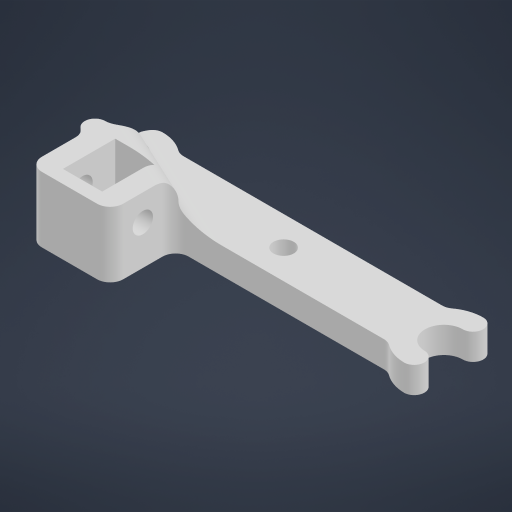
# Autodesk Inventor part: BaseMount
Saved by Autodesk Inventor 2023 (Build 270158000, 158)
## iProperties
Created: 2023-03-14
Part Number: BaseMount
Material: Generic
Document SubType Name: Modeling
Designer: Matt
Density: 1 g/cm^3
Appearance: Default
Author: Matt
Autodesk Inventor part; units mm, degrees
ref_plane "YZ Plane" through (0, 0, 0) normal (1, 0, 0) x (0, 1, 0)
ref_plane "XZ Plane" through (0, 0, 0) normal (0, 1, 0) x (-1, 0, 0)
ref_plane "XY Plane" through (0, 0, 0) normal (0, 0, 1) x (1, 0, 0)
sketch "Sketch1" plane through (0, 0, 0) normal (0, 1, 0) x (-1, 0, 0)
  circle A0 centre (0, 0) radius 2.4868
  line L0 (2.8868, 0) -> (1.4434, 2.5)
  line L1 (1.4434, 2.5) -> (-1.4434, 2.5)
  line L2 (-1.4434, 2.5) -> (-2.8868, 0)
  line L3 (-2.8868, 0) -> (-1.4434, -2.5)
  line L4 (-1.4434, -2.5) -> (1.4434, -2.5)
  line L5 (1.4434, -2.5) -> (2.8868, 0)
  line L6 (0, 0) -> (-23.467, 0)
  circle A1 centre (-49, 0) radius 2.4868
  line L7 (-46.1132, 0) -> (-47.5566, 2.5)
  line L8 (-47.5566, 2.5) -> (-50.4434, 2.5)
  line L9 (-50.4434, 2.5) -> (-51.8868, 0)
  line L10 (-51.8868, 0) -> (-50.4434, -2.5)
  line L11 (-50.4434, -2.5) -> (-47.5566, -2.5)
  line L12 (-47.5566, -2.5) -> (-46.1132, 0)
  arc A2 (43.788, 27) -> (35.788, 35) centre (35.788, 27) ccw
  line L13 (35.788, 35) -> (-48.212, 35)
  arc A3 (-48.212, 35) -> (-56.212, 27) centre (-48.212, 27) ccw
  line L14 (-56.212, 27) -> (-56.212, -62.0882)
  arc A4 (-56.212, -62.0882) -> (-54.3404, -67.2305) centre (-48.212, -62.0882) ccw
  line L15 (-54.3404, -67.2305) -> (-37.6324, -87.1423)
  arc A5 (-37.6324, -87.1423) -> (-31.504, -90) centre (-31.504, -82) ccw
  line L16 (-31.504, -90) -> (19.08, -90)
  arc A6 (19.08, -90) -> (25.2084, -87.1423) centre (19.08, -82) ccw
  line L17 (25.2084, -87.1423) -> (41.9164, -67.2305)
  arc A7 (41.9164, -67.2305) -> (43.788, -62.0882) centre (35.788, -62.0882) ccw
  line L18 (43.788, -62.0882) -> (43.788, 27)
  arc A8 (-17.212, -66) -> (-11.212, -72) centre (-11.212, -66) ccw
  line L19 (-11.212, -72) -> (-1.212, -72)
  arc A9 (-1.212, -72) -> (4.788, -66) centre (-1.212, -66) ccw
  line L20 (4.788, -66) -> (4.788, -64)
  arc A10 (10.788, -58) -> (4.788, -64) centre (10.788, -64) ccw
  line L21 (10.788, -58) -> (25.4731, -58)
  arc A11 (29.3447, -59.4162) -> (25.4731, -58) centre (25.4731, -64) ccw
  line L22 (29.3447, -59.4162) -> (31.3866, -61.1409)
  arc A12 (32.1113, -69.5814) -> (31.3866, -61.1409) centre (27.515, -65.7247) ccw
  line L23 (32.1113, -69.5814) -> (21.8111, -81.8567)
  arc A13 (17.2148, -84) -> (21.8111, -81.8567) centre (17.2148, -78) ccw
  line L24 (17.2148, -84) -> (-29.6388, -84)
  arc A14 (-34.2351, -81.8567) -> (-29.6388, -84) centre (-29.6388, -78) ccw
  line L25 (-34.2351, -81.8567) -> (-44.5353, -69.5814)
  arc A15 (-43.8106, -61.1409) -> (-44.5353, -69.5814) centre (-39.939, -65.7247) ccw
  line L26 (-43.8106, -61.1409) -> (-41.7687, -59.4162)
  arc A16 (-37.8971, -58) -> (-41.7687, -59.4162) centre (-37.8971, -64) ccw
  line L27 (-37.8971, -58) -> (-23.212, -58)
  arc A17 (-17.212, -64) -> (-23.212, -58) centre (-23.212, -64) ccw
  line L28 (-17.212, -64) -> (-17.212, -66)
  circle A18 centre (0, -58) radius 1.375
  circle A19 centre (0, 0) radius 1.5
  circle A20 centre (-49, -58) radius 1.375
  circle A21 centre (-51.962, 9) radius 0.575
  circle A22 centre (39.538, 27) radius 0.575
  circle A23 centre (39.538, 9) radius 0.575
  circle A24 centre (36.576, 0) radius 1.5
  circle A25 centre (36.576, -43.18) radius 1.5
  circle A26 centre (0, -43.18) radius 1.5
  circle A27 centre (-49, 0) radius 1.375
  circle A28 centre (-51.962, 27) radius 0.575
  circle A29 centre (-6.212, -53.538) radius 1.15
  circle A30 centre (-6.212, -67) radius 1.15
  line L29 (35.788, 35) -> (-48.212, 35)
  line L30 (-6.212, 35) -> (-6.212, -103.5846)
  dimension "d2" = 49
  constraints: 62 end point, 32 point on circle, 31 centre point, 2 horizontal, 1 collinear, 1 midpoint, 1 tangent, 1 vertical, 16 other
  measures "d2" distance of point (0, 0) point (-49, 0)
sketch "Sketch2" plane through (0, 0, 0) normal (0, 1, 0) x (-1, 0, 0)
  line L0 (-2.8868, 0) -> (-1.4434, -2.5) projected
  line L1 (1.4434, -2.5) -> (2.8868, 0) projected
  circle A0 centre (0, 0) radius 2.8868
  circle A1 centre (0, 0) radius 6
  arc A2 (0, -6) -> (0, -2.8868) centre (0, -4.4434) ccw
  arc A3 (0, 2.8868) -> (0, 6) centre (-0.1105, 4.4434) ccw
  line L2 (0, -4.4434) -> (-24.5, -4.4434)
  line L3 (-24.5, -4.4434) -> (-24.5, 4.4434)
  line L4 (-24.5, 4.4434) -> (0, 4.4434)
  line L5 (0, 4.4434) -> (0, -4.4434)
  line L6 (-46.1132, 0) -> (-47.5566, -2.5)
  line L7 (-50.4434, -2.5) -> (-51.8868, 0)
  circle A4 centre (-49, 0) radius 2.8868
  circle A5 centre (-49, 0) radius 6
  arc A6 (-49, -2.8868) -> (-49, -6) centre (-49, -4.4434) ccw
  arc A7 (-49, 6) -> (-49, 2.8868) centre (-48.8895, 4.4434) ccw
  line L8 (-49, -4.4434) -> (-24.5, -4.4434)
  line L9 (-24.5, 4.4434) -> (-49, 4.4434)
  line L10 (-49, 4.4434) -> (-49, -4.4434)
  circle A8 centre (-24.5, 0) radius 1.55
  line L11 (-6.212, 35) -> (-6.212, -103.5846) projected
  line L12 (0, 4.4434) -> (-12.424, 4.4434)
  line L13 (-12.424, 4.4434) -> (-12.424, 14.4434)
  line L14 (-12.424, 14.4434) -> (0, 14.4434)
  line L15 (0, 14.4434) -> (0, 4.4434)
  line L16 (-12.424, 4.4434) -> (-2.8868, 4.4434)
  line L17 (-2.8868, 4.4434) -> (-2.8868, 0)
  line L18 (-2.8868, 0) -> (-12.424, 0)
  line L19 (-12.424, 0) -> (-12.424, 4.4434)
  line L20 (-6.212, 4.4434) -> (-3.212, 4.4434)
  line L21 (-3.212, 4.4434) -> (-3.212, 12.4434)
  line L22 (-3.212, 12.4434) -> (-6.212, 12.4434)
  line L23 (-6.212, 12.4434) -> (-6.212, 4.4434)
  line L24 (-6.212, 4.4434) -> (-9.212, 4.4434)
  line L25 (-9.212, 4.4434) -> (-9.212, 12.4434)
  line L26 (-9.212, 12.4434) -> (-6.212, 12.4434)
  line L27 (-12.424, 4.4434) -> (-2.8868, 0)
  point P0 (0, 0)
  point P1 (-4.0319, -4.4434)
  point P2 (-4.0319, 4.4434)
  point P3 (-44.9681, 4.4434)
  point P4 (-44.9681, -4.4434)
  point P5 (0, 6)
  point P6 (0, 6)
  point P7 (-9.5372, 4.4434)
  point P8 (-3.212, 5.0678)
  dimension "d7" = 12
  dimension "d9" = 3.1
  dimension "d14" = 12.424
  dimension "d15" = 10
  dimension "d16" = 6.212
  dimension "d24" = 3
  dimension "d25" = 8
  constraints: 50 end point, 18 point on circle, 9 centre point, 8 parallel, 4 horizontal, 4 perpendicular, 3 symmetric about line, 2 coincident, 2 point on line, 2 tangent, 1 midpoint
  measures "d7" diameter of A1
  measures "d9" diameter of A8
  measures "d14" distance of L13.end L14.end
  measures "d15" distance of L12.end L13.end
  measures "d16" distance between parallel lines of L15 L11
  measures "d24" distance of L22.end L21.end
  measures "d25" distance of L21.end L20.end
extrude "Extrusion1" add sketch "Sketch2" along normal blind 4 contours L17 L4 L5 A0 | L27 A1 L4 L17 | A0 L5 L2 A1 L18 | L18 A1 L27 | L5 L15 A3 | L4 L21 A1 L15 | L18 L11 L27 A1 | A1 L2 L11 L18 | L27 L11 L4 A1 | A2 A1 L2 L5 | L18 L19 L27 L11 | L11 L2 L3 A8 L4 L19 L18 | L27 L4 L11 | L8 A5 L9 L3 A8 | L8 L10 A4 L9 A5 | A5 A6 L10 L8 | L9 L10 A7 A5
extrude "Extrusion3" add sketch "Sketch2" along normal blind 10 contours L17 L4 L5 A0 | L27 A1 L4 L17 | L5 L15 A3 | L4 L21 A1 L15 | L27 L11 L4 A1 | A1 L21 L22 L11 L14 L15 | L27 L4 L11 | L13 L14 L11 L26 L25 L4
sketch "Sketch4" plane through (12.424, 0, 14.4434) normal (1, 0, 0) x (0, 0, -1)
  line L0 (2, 0) -> (2, 10) projected
  line L1 (2, 10) -> (10, 10)
  line L2 (10, 10) -> (10, 0)
  line L3 (10, 0) -> (2, 0)
  line L4 (2, 0) -> (2, 10)
  circle A0 centre (5, 6) radius 1.55
  point P0 (14.4434, 0)
  dimension "d26" = 8
  dimension "d27" = 3.1
  dimension "d28" = 4
  dimension "d31" = 3
  constraints: 8 end point, 2 parallel, 1 centre point, 1 horizontal, 1 perpendicular
  measures "d26" distance of L2.end L3.end
  measures "d27" diameter of A0
  measures "d28" distance from line of L1 A0.centre
  measures "d31" distance from line of L0 A0.centre
extrude "Extrusion4" cut sketch "Sketch4" against normal up to surface (12.424 mm away) contours A0
fillet "Fillet3" radius 3 2 edges at (7.6554, 4, 2.2217) (7.6554, 10, 2.2217)
fillet "Fillet3" radius 2 7 edges at (12.424, 2, 4.4434) (12.424, 5, 14.4434) (0, 5, 14.4434) (44.9681, 2, 4.4434) (44.9681, 2, -4.4434) (4.0319, 2, -4.4434) (0, 5, 6)
equation "\"d14\" = 2 * d16"
equation "\"d24\" = Acrylic"
equation "\"Acrylic\" = 3"
body "Solid1"
